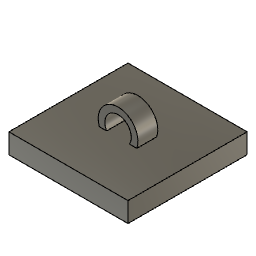
wire hook (Autodesk Fusion 360 design; units mm, degrees)
Autodesk Fusion 360 part; units mm, degrees
sketch "Sketch1" plane through (0, 0, 0) normal (0, 0, 1) x (1, 0, 0)
  line L0 (9, 9) -> (-9, 9)
  line L1 (-9, 9) -> (-9, -9)
  line L2 (-9, -9) -> (9, -9)
  line L3 (9, -9) -> (9, 9)
  line L4 (9, 9) -> (-9, -9) construction
  line L5 (-9, 9) -> (9, -9) construction
  dimension "d1" = 18
  dimension "d2" = 18
  constraint horizontal L0
  constraint perpendicular L0 L1
  constraint parallel L0 L2
  constraint parallel L1 L3
  constraint coincident L4 origin
  constraint coincident L5 origin
  measures "d1" distance of L1.end L2.end
  measures "d2" distance of L0.end L1.end
extrude "Extrude1" add sketch "Sketch1" along normal blind 3
sketch "Sketch3" plane through (0, 0, 0) normal (0, 1, 0) x (1, 0, 0)
  circle A0 centre (0, -4) radius 3
  circle A1 centre (0, -4) radius 2
  dimension "d5" = 6
  dimension "d6" = 4
  constraint concentric A0 A1
  measures "d5" diameter of A0
  measures "d6" diameter of A1
extrude "Extrude2" add sketch "Sketch3" along normal mid plane 3
